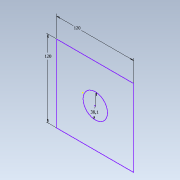
# Autodesk Inventor part: placa inferior
Saved by Autodesk Inventor 2021 (Build 250183000, 183)
## iProperties
Created: 2021-08-20
Part Number: placa inferior
Material: Generic
Document SubType Name: Modeling
Designer: Andrés Holguín
Density: 1 g/cm^3
Appearance: Default
Author: Andrés Holguín
Autodesk Inventor part; units mm, degrees
ref_plane "YZ Plane" through (0, 0, 0) normal (1, 0, 0) x (0, 1, 0)
ref_plane "XZ Plane" through (0, 0, 0) normal (0, 1, 0) x (-1, 0, 0)
ref_plane "XY Plane" through (0, 0, 0) normal (0, 0, 1) x (1, 0, 0)
sketch "Sketch1" plane through (0, 0, 0) normal (0, 0, 1) x (1, 0, 0)
  line L0 (-40.7788, 51.9292) -> (79.2212, 51.9292)
  line L1 (79.2212, 51.9292) -> (79.2212, -68.0708)
  line L2 (79.2212, -68.0708) -> (-40.7788, -68.0708)
  line L3 (-40.7788, -68.0708) -> (-40.7788, 51.9292)
  circle A0 centre (19.2212, -8.0708) radius 19.05
  point P0 (0, 0)
  dimension "d0" = 120
  dimension "d1" = 120
  dimension "d2" = 38.1
  constraints: 8 end point, 2 parallel, 1 centre point, 1 horizontal, 1 perpendicular
  measures "d0" distance of L2.end L0.start
  measures "d1" distance of L0.start L0.end
  measures "d2" diameter of A0
extrude "Extrusion1" add sketch "Sketch1" along normal blind 12.7
sketch "Sketch2" plane through (0, 0, 12.7) normal (0, 0, 1) x (1, 0, 0)
  line L0 (-40.7788, 51.9292) -> (-40.7788, -68.0708) projected
  line L1 (-40.7788, -8.0708) -> (79.2212, -8.0708)
  line L2 (79.2212, -68.0708) -> (79.2212, 51.9292) projected
  line L3 (79.2212, 51.9292) -> (-40.7788, 51.9292) projected
  line L4 (19.2212, 51.9292) -> (19.2212, -68.0708)
  line L5 (-40.7788, -68.0708) -> (79.2212, -68.0708) projected
  point P0 (0, 0)
  point P1 (-25.2788, 36.4292)
  point P2 (63.7212, 36.4292)
  point P3 (63.7212, -52.5708)
  point P4 (-25.2788, -52.5708)
  dimension "d5" = 89
  dimension "d6" = 89
  dimension "d7" = 89
  dimension "d8" = 89
  constraints: 4 end point, 4 midpoint, 2 symmetric about line
  measures "d5" distance of point (-25.279, 36.429) point (63.721, 36.429)
  measures "d6" distance of point (-25.279, -52.571) point (-25.279, 36.429)
  measures "d7" distance of point (63.721, 36.429) point (63.721, -52.571)
  measures "d8" distance of point (-25.279, -52.571) point (63.721, -52.571)
hole "Hole1" at (-25.2788, 36.4292, 12.7) at (63.7212, 36.4292, 12.7) at (63.7212, -52.5708, 12.7) at (-25.2788, -52.5708, 12.7) direction (0, 0, -1) diameter 10 end through all
body "Solid1"
